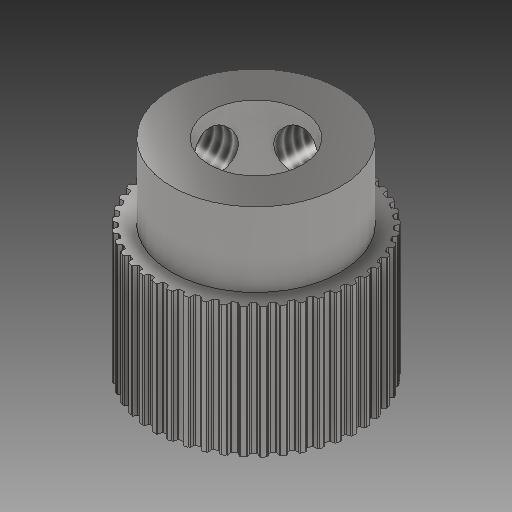
# Autodesk Inventor part: Extruder Knob
Saved by Autodesk Inventor 2020.2 (Build 242310000, 310)
## iProperties
Created: 2020-03-05
Part Number: Extruder Knob
Material: Stainless Steel
Document SubType Name: Modeling
Designer: Richard Hall
Density: 8 g/cm^3
Appearance: Semi-Polished
Author: Richard Hall
Title: 11mm Extruder Knob
Autodesk Inventor part; units mm, degrees
ref_plane "YZ Plane" through (0, 0, 0) normal (1, 0, 0) x (0, 1, 0)
ref_plane "XZ Plane" through (0, 0, 0) normal (0, 1, 0) x (-1, 0, 0)
sketch "Sketch1" plane through (0, 0, 0) normal (0, 1, 0) x (-1, 0, 0)
  circle A0 centre (0, 0) radius 5.4737
  circle A1 centre (0, 0) radius 2.5
  dimension "d0" = 10.9474
  dimension "d1" = 5
  constraints: 2 centre point, 2 coincident
  measures "d0" diameter of A0
  measures "d1" diameter of A1
extrude "Extrusion1" add sketch "Sketch1" along normal blind 10.9855
ref_plane "Work Plane1" through (0, 7, 0) normal (0, -1, 0) x (1, 0, 0)
sketch "Sketch2" plane through (0, 10.9855, 0) normal (0, 1, 0) x (1, 0, 0)
  circle A0 centre (0, 0) radius 5.4737 projected
  circle A1 centre (0, 0) radius 4.5339
  dimension "d4" = 9.0678
  constraints: 1 centre point, 1 coincident
  measures "d4" diameter of A1
extrude "Extrusion2" cut sketch "Sketch2" against normal up to surface (3.9855 mm away)
sketch "Sketch3" plane through (0, 7, 0) normal (0, 1, 0) x (1, 0, 0)
  line L0 (0, 0) -> (-0.3818, 5.4594)
  line L1 (0, 0) -> (0.3818, 5.4594)
  line L2 (-0.3818, 5.4594) -> (-0.282, 5.4664)
  arc A0 (-0.2245, 5.4308) -> (-0.282, 5.4664) centre (-0.278, 5.4087) ccw
  line L3 (-0.2245, 5.4308) -> (-0.1535, 5.2594)
  arc A1 (-0.1535, 5.2594) -> (-0.1, 5.2237) centre (-0.1, 5.2816) ccw
  line L4 (-0.1, 5.2237) -> (0.1, 5.2237)
  arc A2 (0.1, 5.2237) -> (0.1535, 5.2594) centre (0.1, 5.2816) ccw
  line L5 (0.1535, 5.2594) -> (0.2245, 5.4308)
  arc A3 (0.282, 5.4664) -> (0.2245, 5.4308) centre (0.278, 5.4087) ccw
  line L6 (0.282, 5.4664) -> (0.3818, 5.4594)
  circle A4 centre (0, 0) radius 5.4737 projected
  point P0 (0, 5.2237)
  point P1 (0.2809, 5.4665)
  point P2 (-0.2809, 5.4665)
  dimension "d7" = 8
  dimension "d8" = 0.1
  dimension "d9" = 0.2
  dimension "d11" = 45
  dimension "d18" = 0.25
  constraints: 14 end point, 8 point on circle, 8 tangent, 4 centre point, 3 equal radius, 2 perpendicular, 1 equal length, 1 horizontal, 1 horizontal alignment, 1 midpoint, 1 vertical alignment, 3 other
  measures "d7" angle of L1 L0
  measures "d8" distance of L0.end L2.end
  measures "d9" distance of L4.start L4.end
  measures "d11" angle of L5 L3
extrude "Extrusion3" cut sketch "Sketch3" against normal blind 10 contours A4 A3 L5 A2 L4 A1 L3 A0
pattern_circular "Circular Pattern1" count 45 over 360 about axis through (0, 10.9855, 0) along (0, -1, 0) of "Extrusion3"
sketch "Sketch4" plane through (0, 0, 0) normal (1, 0, 0) x (0, 1, 0)
  line L0 (10.9855, -4.5339) -> (10.9855, 4.5339) projected
  line L1 (7, -5.0134) -> (7, -5.1586) projected
  line L2 (7, -5.0134) -> (10.9855, -5.0134)
  point P0 (0, 0)
  point P1 (7, -5.0526)
  point P2 (8.9928, 0)
  point P3 (8.9928, -5.0134)
  point P4 (10.9855, 0)
  constraints: 2 end point, 2 midpoint, 1 horizontal, 1 horizontal alignment, 1 point on line, 1 vertical alignment
hole "Hole1" at (0, 8.9928, 0) direction (-1, 0, 0) diameter 2.459 end through all thread size "M3x0.5" class "6H" standard "ANSI Metric M Profile"
pattern_circular "Circular Pattern2" count 2 over 90 about axis through (0, 10.9855, 0) along (0, -1, 0) of "Hole1"
equation "\"d9\" = 2 * d8"
body "Solid1"
